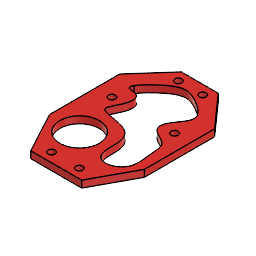
Simple gripper_palm (Autodesk Fusion 360 design; units mm, degrees)
Autodesk Fusion 360 part; units mm, degrees
sketch "Sketch1" plane through (0, 0, 0) normal (0, 0, 1) x (1, 0, 0)
  line L0 (51, 21.4003) -> (51, -40.5997)
  line L1 (51, 21.4003) -> (58.9898, 21.4003)
  line L2 (58.9898, 21.4003) -> (71.5, 7.3)
  line L3 (71.5, 7.3) -> (71.5, -23)
  line L4 (71.5, -23) -> (62, -40.5997)
  line L5 (62, -40.5997) -> (51, -40.5997)
  circle A0 centre (56.2398, 17.4003) radius 1.5
  circle A1 centre (64.5, -3) radius 1.5
  circle A2 centre (57, -36.5997) radius 1.5
  circle A3 centre (45, -36.5997) radius 1.5
  line L6 (40, -40.5997) -> (51, -40.5997)
  circle A4 centre (45.7602, 17.4003) radius 1.5
  line L7 (30.5, -23) -> (40, -40.5997)
  line L8 (30.5, 7.3) -> (30.5, -23)
  circle A5 centre (37.5, -3) radius 1.5
  line L9 (51, 21.4003) -> (43.0102, 21.4003)
  line L10 (51, 21.4003) -> (51, -40.5997)
  line L11 (43.0102, 21.4003) -> (30.5, 7.3)
  circle A6 centre (43.5, -23) radius 8.5
  line L12 (30.5, -23) -> (51, -23) construction
  spline S0 degree 5 poles (38, 6) (38.1304, 6.2316) (38.4362, 6.7206) (39.0212, 7.5237) (40.0163, 8.6973) (41.5112, 10.2331) (43.1479, 11.7302) (44.8275, 13.0851) (46.4731, 14.2072) (48.0406, 15.0263) (49.5346, 15.5029) (50.9992, 15.6286) (52.4924, 15.4186) (54.0641, 14.9071) (55.7354, 14.1419) (57.4709, 13.1785) (59.1786, 12.0754) (60.7383, 10.8876) (62.0212, 9.6618) (62.9141, 8.4305) (63.3396, 7.207) (63.283, 5.9774) (62.7929, 4.7093) (61.9678, 3.3689) (60.9476, 1.9361) (59.9033, 0.4203) (59.0263, -1.1257) (58.4974, -2.6268) (58.4565, -4.006) (58.9727, -5.2045) (60.0113, -6.2031) (61.4125, -7.0383) (62.9513, -7.7817) (64.3901, -8.5222) (65.5323, -9.348) (66.279, -10.3281) (66.6744, -11.4953) (66.8447, -12.8547) (66.9409, -14.3888) (67.0863, -16.0645) (67.3091, -17.8393) (67.5458, -19.6648) (67.6847, -21.487) (67.5958, -23.2481) (67.1671, -24.8873) (66.3368, -26.3422) (65.1312, -27.5498) (63.6442, -28.4508) (62.0105, -28.9936) (60.3815, -29.1389) (58.9004, -28.8635) (57.675, -28.1657) (56.7688, -27.0658) (56.1982, -25.6068) (55.9281, -23.854) (55.8673, -21.896) (55.8668, -19.8438) (55.7513, -17.8171) (55.3473, -15.9316) (54.513, -14.2857) (53.1673, -12.9481) (51.3189, -11.9444) (49.0965, -11.2437) (46.7096, -10.7728) (44.4076, -10.4303) (42.4393, -10.1009) (41.0111, -9.6697) (40.2502, -9.0362) (40.1538, -8.13) (40.5883, -6.9198) (41.3451, -5.419) (42.1818, -3.6895) (42.8708, -1.8497) (43.2392, -0.0719) (43.1757, 1.4642) (42.6444, 2.6148) (41.6924, 3.3108) (40.4679, 3.6114) (39.2069, 3.7079) (38.1609, 3.8328) (37.5433, 4.1974) (37.4723, 4.7604) (37.6536, 5.331) (37.8696, 5.7684) (38, 6) knots 0 0 0 0 0 0 0.0125 0.025 0.0375 0.05 0.0625 0.075 0.0875 0.1 0.1125 0.125 0.1375 0.15 0.1625 0.175 0.1875 0.2 0.2125 0.225 0.2375 0.25 0.2625 0.275 0.2875 0.3 0.3125 0.325 0.3375 0.35 0.3625 0.375 0.3875 0.4 0.4125 0.425 0.4375 0.45 0.4625 0.475 0.4875 0.5 0.5125 0.525 0.5375 0.55 0.5625 0.575 0.5875 0.6 0.6125 0.625 0.6375 0.65 0.6625 0.675 0.6875 0.7 0.7125 0.725 0.7375 0.75 0.7625 0.775 0.7875 0.8 0.8125 0.825 0.8375 0.85 0.8625 0.875 0.8875 0.9 0.9125 0.925 0.9375 0.95 0.9625 0.975 0.9875 1 1 1 1 1 1
  point P0 (47.1022, 14.5001)
  point P1 (54.9014, 14.5001)
  point P2 (63, 8)
  point P3 (61, 2)
  point P4 (59, -5)
  point P5 (65.3423, -9.2997)
  point P6 (67, -15)
  point P7 (67, -25)
  point P8 (60, -29)
  point P9 (56, -24)
  point P10 (53, -13)
  point P11 (40.6867, -9.2997)
  point P12 (42, -4)
  point P13 (42, 3)
  point P14 (38, 4)
  dimension "d1" = 62
  dimension "d2" = 18.85
  dimension "d3" = 30.3
  dimension "d4" = 20
  dimension "d5" = 11
  dimension "d6" = 20.5
  dimension "d7" = 3
  dimension "d8" = 3
  dimension "d9" = 3
  dimension "d10" = 2.75
  dimension "d11" = 4
  dimension "d12" = 7
  dimension "d13" = 10.3
  dimension "d14" = 4
  dimension "d15" = 6
  dimension "d16" = 17
  dimension "d17" = 13
  constraint vertical L0
  constraint perpendicular L0 L1
  constraint perpendicular L1 L3
  constraint perpendicular L0 L5
  constraint symmetric L1.start L0 L9.start
  constraint symmetric L5.end L0 L6.end
  constraint symmetric L0 L1.end L9.end
  constraint symmetric L0 L2.end L8.start
  constraint symmetric L0 L3.end L7.start
  constraint symmetric L0 L4.end L6.start
  constraint symmetric L0 A0 A4
  constraint symmetric L0 A1 A5
  constraint symmetric L0 A2 A3
  constraint coincident L0 L12.end
  constraint perpendicular L0 L12
  constraint coincident A6.centre L12
  measures "d1" distance of L0.start L0.end
  measures "d2" distance of L1.end L2.end
  measures "d3" distance of L2.end L3.end
  measures "d4" distance of L3.end L4.end
  measures "d5" distance of L0.end L4.end
  measures "d6" distance of L0 L3
  measures "d7" diameter of A0
  measures "d8" diameter of A1
  measures "d9" diameter of A2
  measures "d10" horizontal distance of L1.end A0.centre
  measures "d11" distance of L1 A0.centre
  measures "d12" distance of L3 A1.centre
  measures "d13" vertical distance of L2.end A1.centre
  measures "d14" distance of L5 A2.centre
  measures "d15" distance of L0 A2.centre
  measures "d16" diameter of A6
  measures "d17" distance of L8 A6.centre
extrude "Extrude1" add sketch "Sketch1" along normal blind 3 contours L0 L1 L2 L3 L4 L5 L10 A6 S0 | L0 L6 L7 L8 L9 L10 L11 A6 S0
